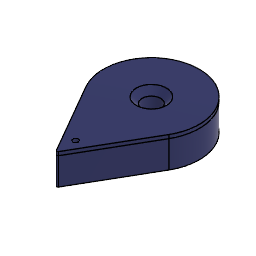
Mini humidifer case_Drop (Autodesk Fusion 360 design; units mm, degrees)
Autodesk Fusion 360 part; units mm, degrees
sketch "Sketch1" plane through (0, 0, 0) normal (0, 0, 1) x (1, 0, 0)
  circle A0 centre (0, 0) radius 10.25
  circle A1 centre (0, 0) radius 13.25
  line L0 (-2.5, -7.9748) -> (2.5, -7.9748)
  line L1 (2.5, -7.9748) -> (2.5, -15.1793)
  line L2 (2.5, -15.1793) -> (-2.5, -15.1793)
  line L3 (-2.5, -15.1793) -> (-2.5, -7.9748)
  circle A2 centre (0, 0) radius 4
  line L4 (9.5, -20) -> (9.5, -55)
  line L5 (9.5, -55) -> (-9.5, -55)
  line L6 (-9.5, -55) -> (-9.5, -20)
  line L7 (-9.5, -20) -> (9.5, -20)
  line L8 (9.5, -20) -> (-9.5, -55) construction
  line L9 (9.5, -55) -> (-9.5, -20) construction
  line L10 (0, 0) -> (0, -75)
  line L11 (0.0866, -74.85) -> (32.476, -18.75)
  line L12 (-0.0866, -74.85) -> (-32.476, -18.75)
  arc A3 (-0.0866, -74.85) -> (0.0866, -74.85) centre (0, -74.8) ccw
  circle A4 centre (0, 0) radius 40.5
  line L13 (0, 0) -> (0, -81)
  line L14 (-32.476, -18.75) -> (-35.074, -20.25)
  line L15 (32.476, -18.75) -> (35.074, -20.25)
  line L16 (35.074, -20.25) -> (0.866, -79.5)
  line L17 (-0.866, -79.5) -> (-35.074, -20.25)
  arc A5 (-0.866, -79.5) -> (0.866, -79.5) centre (0, -79) ccw
  circle A6 centre (0, -64) radius 2.25
  circle A7 centre (0, 0) radius 5
  circle A8 centre (32.9, -0.01) radius 4.6
  circle A9 centre (32.9, -0.01) radius 1.6
  line L18 (32.9, 4.59) -> (37.218, 4.59)
  line L19 (37.2156, -4.61) -> (32.9, -4.61)
  circle A10 centre (-32.9, 0.0531) radius 4.6
  circle A11 centre (-32.9, 0.0531) radius 1.6
  line L20 (-32.9, 4.6531) -> (-37.2102, 4.6531)
  line L21 (-32.9, -4.5469) -> (-37.2233, -4.5469)
  circle A12 centre (0, 0) radius 37
  line L22 (0, 0) -> (0, -74)
  line L23 (-1.299, -71.75) -> (-32.0429, -18.5)
  line L24 (1.299, -71.75) -> (32.0429, -18.5)
  arc A13 (-1.299, -71.75) -> (1.299, -71.75) centre (0, -71) ccw
  circle A14 centre (0, 0) radius 34
  line L25 (0, 0) -> (0, -68)
  line L26 (0, -68) -> (-29.4449, -17)
  line L27 (0, -68) -> (29.4449, -17)
  circle A15 centre (0, -64) radius 2.75
  circle A16 centre (0, 0) radius 7.75
  circle A17 centre (0, 0) radius 10
  arc A18 (32.476, -18.75) -> (-32.476, -18.75) centre (0, 0) ccw
  line L28 (-1.3856, -71.9) -> (-32.1728, -18.575)
  arc A19 (32.1728, -18.575) -> (-32.1728, -18.575) centre (0, 0) ccw
  line L29 (1.3856, -71.9) -> (32.1728, -18.575)
  arc A20 (-1.3856, -71.9) -> (1.3856, -71.9) centre (0, -71.1) ccw
  point P0 (0, -10.25)
  point P1 (0, -37.5)
  dimension "d1" = 20.5
  dimension "d4" = 26.5
  dimension "d8" = 8
  dimension "d9" = 35
  dimension "d10" = 19
  dimension "d12" = 75
  dimension "d13" = 0.1
  dimension "d14" = 81
  dimension "d15" = 81
  dimension "d16" = 1
  dimension "d17" = 4.5
  dimension "d26" = 9.2
  dimension "d27" = 3.2
  dimension "d28" = 9.2
  dimension "d29" = 3.2
  dimension "d33" = 74
  dimension "d34" = 74
  dimension "d35" = 1.5
  dimension "d36" = 68
  dimension "d37" = 68
  dimension "d38" = 5.5
  dimension "d54" = 15.5
  dimension "d60" = 20
  dimension "d69" = 1.6
  constraint coincident A0.centre A1.centre
  constraint concentric A0 A1
  constraint coincident A0 P0
  constraint horizontal L0
  constraint vertical L1
  constraint horizontal L2
  constraint vertical L3
  constraint perpendicular L4 L5
  constraint parallel L4 L6
  constraint parallel L5 L7
  constraint coincident L8 P1
  constraint coincident L9 P1
  constraint coincident L10.end L11
  constraint coincident L10.end L12
  constraint tangent L11 A3
  constraint tangent L12 A3
  constraint parallel L10 L13
  constraint coincident A4 L14.end
  constraint perpendicular L12 L14
  constraint coincident A4 L15.end
  constraint perpendicular L11 L15
  constraint tangent A4 L16
  constraint coincident L13.end L16
  constraint coincident L13.end L17
  constraint tangent L16 A5
  constraint tangent L17 A5
  constraint coincident L10 A6.centre
  constraint concentric A1 A7
  constraint concentric A8 A9
  constraint coincident A8 L18.start
  constraint tangent A8 L18
  constraint horizontal L18
  constraint coincident A8 L19.end
  constraint tangent A8 L19
  constraint concentric A10 A11
  constraint coincident A10 L20.start
  constraint tangent A10 L20
  constraint horizontal L20
  constraint coincident A10 L21.start
  constraint tangent A10 L21
  constraint parallel L20 L21
  constraint concentric A1 A12
  constraint parallel L10 L22
  constraint coincident A12 L23.end
  constraint tangent A12 L23
  constraint coincident A12 L24.end
  constraint tangent A12 L24
  constraint coincident L22.end L24
  constraint coincident L22.end L23
  constraint tangent L24 A13
  constraint tangent L23 A13
  constraint concentric A12 A14
  constraint parallel L10 L25
  constraint coincident A14 L26.end
  constraint tangent A14 L26
  constraint coincident A14 L27.end
  constraint tangent A14 L27
  constraint concentric A6 A15
  constraint concentric A4 A16
  constraint concentric A12 A17
  constraint concentric A18 A19
  constraint tangent L28 A19
  constraint tangent A19 L29
  constraint tangent L28 A20
  constraint tangent L29 A20
  measures "d1" diameter of A0
  measures "d4" diameter of A1
  measures "d8" diameter of A2
  measures "d9" distance of L5.end L6.end
  measures "d10" distance of L4.end L5.end
  measures "d12" distance of A0.centre L10.end
  measures "d13" radius of A3
  measures "d14" diameter of A4
  measures "d15" distance of A0.centre L13.end
  measures "d16" radius of A5
  measures "d17" diameter of A6
  measures "d26" diameter of A8
  measures "d27" diameter of A9
  measures "d28" diameter of A10
  measures "d29" diameter of A11
  measures "d33" diameter of A12
  measures "d34" distance of A0.centre L22.end
  measures "d35" radius of A13
  measures "d36" diameter of A14
  measures "d37" distance of A0.centre L25.end
  measures "d38" diameter of A15
  measures "d54" diameter of A16
  measures "d60" diameter of A17
  measures "d69" radius of A20
extrude "Extrude2" add sketch "Sketch1" along normal blind 3 contours A0 L1 L3 A17 | A0 A1 L1 L3 | A0 L3 L10 L13 L22 L25 A17 | A0 A1 L3 L10 L13 L22 L25 | A0 A1 L1 L10 L13 L22 L25 | A0 L1 L10 L13 L22 L25 A17 | A1 L2 L3 L10 L13 L22 L25 | L0 L1 L3 A17 | L0 L3 L10 L13 L22 L25 A17 | L0 L1 L10 L13 L22 L25 A17 | A1 L1 L2 L10 L13 L22 L25 | A2 | L4 L6 L7 A8 L18 L19 A10 L20 L21 A14 | L4 L7 L10 L13 L22 A14 L25 | L4 A12 A14 L27 | L4 L10 L13 A12 L22 A14 L25 | L6 L7 L10 L13 L22 A14 L25 | L4 A4 A12 L27 | L4 L10 A4 L13 A12 L22 L25 | L6 L10 L13 A12 L22 A14 L25 | L19 A12 A14 L27 | L4 A4 L27 | L4 L5 L10 A4 L13 L22 L25 L27 | L6 L10 A4 L13 A12 L22 L25 | A4 A12 L24 L27 | L6 A12 A14 L26 | A8 L19 A12 A14 | A8 L19 A14 | L4 L5 L10 A4 L13 L22 L24 A13 L27 A15 | L4 L5 L27 | L5 L6 L10 A4 L13 L22 L25 L26 | L6 A4 A12 L26 | A4 L19 A12 L24 A19 L29 | L21 A12 A14 L26 | A8 L19 A12 A19 | A8 A9 A14 | A8 A9 A12 A14 | L5 L10 L13 L22 L25 L27 A15 | L5 L10 L13 L22 L25 L26 A15 | L6 A4 L26 | L10 A4 L13 L22 L24 A13 L29 A20 | A4 A12 L23 L26 | A10 L21 A14 | A10 L21 A12 A14 | A8 L19 A18 A19 | L11 A4 L19 A18 A19 L29 | A8 A12 A19 | A8 L18 A14 | A9 A14 | A9 A14 | A6 L27 A15 | L10 L13 A6 L22 L25 L27 A15 | L5 L6 L10 A4 L13 L22 L23 A13 L26 A15 | L5 L6 L26 | L10 L13 A6 L22 L25 L26 A15 | L10 L11 A3 A4 L13 L22 L29 A20 | A4 L21 A12 L23 L28 A19 | A10 A11 A14 | A10 L21 A12 A19 | A10 A11 A12 A14 | A4 L14 L15 A18 | A8 A19 | A8 L18 A12 A14 | L18 L20 A12 A14 | L10 L13 A6 L22 L25 L27 | A6 L27 | A6 L26 A15 | L10 L13 A6 L22 L25 L26 | L10 A4 L13 L22 L23 A13 L28 A20 | L10 L11 A3 A4 L13 L16 A5 | L11 A4 L15 | L12 A4 L21 A18 L28 A19 | A10 L21 A18 A19 | A10 A12 A19 | A11 A14 | A11 A14 | A8 L18 A18 A19 | A8 L18 A12 A19 | L18 L20 A12 A19 | A10 L20 A12 A14 | A10 L20 A14 | L10 L13 A6 L22 L25 L27 A15 | L10 L13 L22 L25 L27 A15 | A6 L26 | L10 L13 L22 L25 L26 A15 | L10 L13 A6 L22 L25 L26 A15 | L10 L12 A3 A4 L13 L22 L28 A20 | A10 A19 | A10 L20 A12 A19 | L18 L20 A18 A19 | L12 A4 L14 | L10 L12 A3 A4 L13 L17 A5 | A10 L20 A18 A19 | A7 | A16 makes body 1
extrude "Extrude14" cut sketch "Sketch1" along normal blind 12 contours A2 bodies 1
extrude "Extrude3" add sketch "Sketch1" along normal blind 20 from surface at 3 contours L10 A4 L13 L22 L24 A13 L29 A20 | A4 L14 L15 A18 | L10 L11 A3 A4 L13 L16 A5 | L11 A4 L15 | L12 A4 L14 | L10 L12 A3 A4 L13 L17 A5 bodies 1
extrude "Extrude8" add sketch "Sketch1" along normal blind 5 from surface at 6 separate body contours A0 A1 L1 L3 makes body 2
extrude "Extrude9" add sketch "Sketch1" along normal blind 3 from surface at 3 contours A0 L1 L3 A17 | A0 A1 L1 L3 | L0 L1 L3 A17 | A7 | A16 bodies 1 2
extrude "Extrude10" add sketch "Sketch1" along normal blind 10 from surface at 3.5 separate body contours L4 L7 L10 L13 L22 A14 L25 | L4 L10 L13 A12 L22 A14 L25 | L6 L7 L10 L13 L22 A14 L25 | L4 L10 A4 L13 A12 L22 L25 | L6 L10 L13 A12 L22 A14 L25 | L4 L5 L10 A4 L13 L22 L25 L27 | L6 L10 A4 L13 A12 L22 L25 | L4 L5 L27 | L5 L6 L10 A4 L13 L22 L25 L26 | L5 L6 L26 makes body 3
extrude "Extrude12" add sketch "Sketch1" along normal blind 5 from surface at 6.5 separate body contours L0 L1 L3 A17 | L0 L3 L10 L13 L22 L25 A17 | L0 L1 L10 L13 L22 L25 A17 | A2 | A7 | A16 makes body 4
sketch "Sketch2" plane through (0, 0, 11.5) normal (0, 0, 1) x (-1, 0, 0)
  circle A0 centre (0, 0) radius 10
  circle A1 centre (0, 0) radius 7.25
  dimension "d73" = 14.5
  constraint coincident A0.centre A1.centre
  measures "d73" diameter of A1
extrude "Extrude15" cut sketch "Sketch2" against normal blind 2 contours A1 bodies 4
extrude "Extrude16" cut sketch "Sketch2" along normal blind 2 from surface at -5 contours A1 bodies 4
move_body "Move1" bodies 1 to x (1, 0, 0) y (0, 1, 0) z (0, 0, 1) at (-90, 0, 0)
move_body "Move2" bodies 3 to x (1, 0, 0) y (0, 1, 0) z (0, 0, 1) at (-90, 0, 0)
move_body "Move3" bodies 4 to x (1, 0, 0) y (0, 1, 0) z (0, 0, 1) at (-90, 0, 0)
extrude "Extrude4" add sketch "Sketch1" along normal blind 3 separate body contours A0 L1 L3 A17 | A0 A1 L1 L3 | A0 L3 L10 L13 L22 L25 A17 | A0 A1 L3 L10 L13 L22 L25 | A0 A1 L1 L10 L13 L22 L25 | A0 L1 L10 L13 L22 L25 A17 | A1 L2 L3 L10 L13 L22 L25 | L0 L1 L3 A17 | L0 L3 L10 L13 L22 L25 A17 | L0 L1 L10 L13 L22 L25 A17 | A1 L1 L2 L10 L13 L22 L25 | L4 L6 L7 A8 L18 L19 A10 L20 L21 A14 | L4 L7 L10 L13 L22 A14 L25 | L4 A12 A14 L27 | L4 L10 L13 A12 L22 A14 L25 | L6 L7 L10 L13 L22 A14 L25 | L4 A4 A12 L27 | L4 L10 A4 L13 A12 L22 L25 | L6 L10 L13 A12 L22 A14 L25 | L19 A12 A14 L27 | L4 A4 L27 | L4 L5 L10 A4 L13 L22 L25 L27 | L6 L10 A4 L13 A12 L22 L25 | A4 A12 L24 L27 | L6 A12 A14 L26 | A8 L19 A12 A14 | A8 L19 A14 | L4 L5 L10 A4 L13 L22 L24 A13 L27 A15 | L4 L5 L27 | L5 L6 L10 A4 L13 L22 L25 L26 | L6 A4 A12 L26 | A4 L19 A12 L24 A19 L29 | L21 A12 A14 L26 | A8 L19 A12 A19 | A8 A9 A14 | A8 A9 A12 A14 | L5 L10 L13 L22 L25 L27 A15 | L5 L10 L13 L22 L25 L26 A15 | L6 A4 L26 | L10 A4 L13 L22 L24 A13 L29 A20 | A4 A12 L23 L26 | A10 L21 A14 | A10 L21 A12 A14 | A8 L19 A18 A19 | L11 A4 L19 A18 A19 L29 | A8 A12 A19 | A8 L18 A14 | A9 A14 | A9 A14 | A6 L27 A15 | L10 L13 A6 L22 L25 L27 A15 | L5 L6 L10 A4 L13 L22 L23 A13 L26 A15 | L5 L6 L26 | L10 L13 A6 L22 L25 L26 A15 | L10 L11 A3 A4 L13 L22 L29 A20 | A4 L21 A12 L23 L28 A19 | A10 A11 A14 | A10 L21 A12 A19 | A10 A11 A12 A14 | A4 L14 L15 A18 | A8 A19 | A8 L18 A12 A14 | L18 L20 A12 A14 | L10 L13 A6 L22 L25 L27 | A6 L27 | A6 L26 A15 | L10 L13 A6 L22 L25 L26 | L10 A4 L13 L22 L23 A13 L28 A20 | L10 L11 A3 A4 L13 L16 A5 | L11 A4 L15 | L12 A4 L21 A18 L28 A19 | A10 L21 A18 A19 | A10 A12 A19 | A11 A14 | A11 A14 | A8 L18 A18 A19 | A8 L18 A12 A19 | L18 L20 A12 A19 | A10 L20 A12 A14 | A10 L20 A14 | L10 L13 A6 L22 L25 L27 A15 | L10 L13 L22 L25 L27 A15 | A6 L26 | L10 L13 L22 L25 L26 A15 | L10 L13 A6 L22 L25 L26 A15 | L10 L12 A3 A4 L13 L22 L28 A20 | A10 A19 | A10 L20 A12 A19 | L18 L20 A18 A19 | L12 A4 L14 | L10 L12 A3 A4 L13 L17 A5 | A10 L20 A18 A19 makes body 5
extrude "Extrude13" cut sketch "Sketch1" along normal blind 6 contours L10 L13 A6 L22 L25 L27 | A6 L27 | L10 L13 A6 L22 L25 L26 | A6 L26 bodies 5
extrude "Extrude6" add sketch "Sketch1" along normal blind 3 from surface at 3 contours L19 A12 A14 L27 | A4 A12 L24 L27 | A8 L19 A12 A14 | L4 L5 L10 A4 L13 L22 L24 A13 L27 A15 | L4 L5 L27 | A4 L19 A12 L24 A19 L29 | L21 A12 A14 L26 | A8 L19 A12 A19 | A8 A9 A12 A14 | L10 A4 L13 L22 L24 A13 L29 A20 | A4 A12 L23 L26 | A10 L21 A12 A14 | A8 A12 A19 | A9 A14 | L5 L6 L10 A4 L13 L22 L23 A13 L26 A15 | L5 L6 L26 | A4 L21 A12 L23 L28 A19 | A10 L21 A12 A19 | A10 A11 A12 A14 | A8 L18 A12 A14 | L18 L20 A12 A14 | L10 A4 L13 L22 L23 A13 L28 A20 | A10 A12 A19 | A11 A14 | A8 L18 A12 A19 | L18 L20 A12 A19 | A10 L20 A12 A14 | L10 L13 L22 L25 L27 A15 | L10 L13 L22 L25 L26 A15 | A10 L20 A12 A19 picked at (34.1608, -0.2093) picked at (-34.1651, 0.0551) bodies 5
chamfer "Chamfer2" distance 0.5 distance2 3 4 edges at (0, 37.15, 6) (-16.7792, -45.2375, 6) (0, -72.7, 6) (16.7792, -45.2375, 6) measured on face at (21.4312, -32.9801, 6) measured on face at (21.4312, -32.9801, 6) measured on face at (21.4312, -32.9801, 6) measured on face at (21.4312, -32.9801, 6) on bodies 5
extrude "Extrude11" add sketch "Sketch1" along normal blind 11.5 from surface at 3 contours A0 L1 L3 A17 | A0 A1 L1 L3 | A0 L3 L10 L13 L22 L25 A17 | A0 A1 L3 L10 L13 L22 L25 | A0 A1 L1 L10 L13 L22 L25 | A0 L1 L10 L13 L22 L25 A17 | L0 L1 L3 A17 | L0 L3 L10 L13 L22 L25 A17 | L0 L1 L10 L13 L22 L25 A17 bodies 5
chamfer "Chamfer1" distance 5 distance2 5 1 edges at (-7.2255, 2.8025, 0) measured on face at (7.7115, 0.7717, 9.6667) on bodies 5
move_body "Move4" bodies 1 3 4 5 to x (1, 0, 0) y (0, 1, 0) z (0, 0, 1) at (90, 0, 0)
move_body "Move5" bodies 5 to x (-1, 0, 0) y (0, 1, 0) z (0, 0, -1) at (200.4849, 0, 6)
move_body "Move6" bodies 5 to x (1, 0, 0) y (0, 1, 0) z (0, 0, 1) at (-110.4849, 0, 20)
equation "d4 = 20.500 mm + 6 mm"
equation "d14 = 75.000 mm + 6 mm"
equation "d15 = 75.000 mm + 6 mm"
equation "d26 = 6 mm + 3.2 mm"
equation "d28 = 6 mm + 3.2 mm"
equation "d36 = 74.000 mm - 6 mm"
equation "d37 = 74 mm - 6 mm"
equation "d38 = 4.500 mm + 1 mm"
equation "d54 = 20.500 mm - 5 mm"
